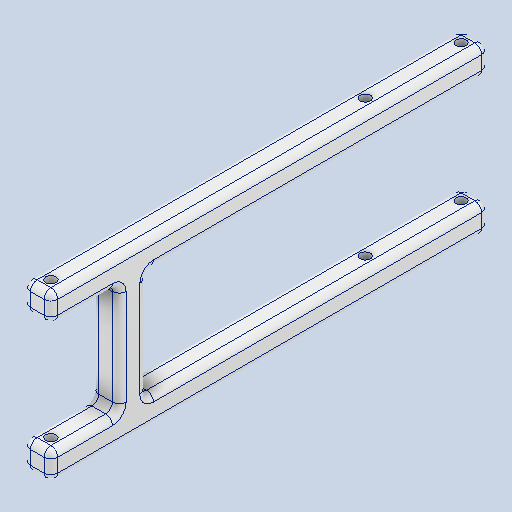
# Autodesk Inventor part: inner swing
Saved by Autodesk Inventor 2023 (Build 270158000, 158)
## iProperties
Created: 2023-01-25
Part Number: inner swing
Material: Aluminum 6061
Document SubType Name: Modeling
Designer: Gabriel - T3 CAD
Density: 2.7 g/cm^3
Appearance: Aluminum - Flat
Mass: 184.405 g
Surface Area: 217.239 cm^2
Volume: 68.2983 cm^3
Author: Gabriel - T3 CAD
Autodesk Inventor part; units mm, degrees
ref_plane "YZ Plane" through (0, 0, 0) normal (1, 0, 0) x (0, 1, 0)
ref_plane "XZ Plane" through (0, 0, 0) normal (0, 1, 0) x (-1, 0, 0)
ref_plane "XY Plane" through (0, 0, 0) normal (0, 0, 1) x (1, 0, 0)
sketch "Sketch1" plane through (0, 0, 0) normal (0, 1, 0) x (-1, 0, 0)
  line L0 (0, 0) -> (12.7, 0)
  line L1 (12.7, 0) -> (12.7, 203.2)
  line L2 (12.7, 203.2) -> (0, 203.2)
  line L3 (0, 203.2) -> (0, 0)
  circle A0 centre (6.35, 6.35) radius 2.3813
  circle A1 centre (6.35, 196.85) radius 2.3813
  circle A2 centre (6.35, 50.8) radius 2.3813
  dimension "d0" = 12.7
  dimension "d1" = 203.2
  dimension "d2" = 6.35
  dimension "d3" = 6.35
  dimension "d4" = 4.7625
  dimension "d5" = 6.35
  dimension "d6" = 4.7625
  dimension "d7" = 6.35
  dimension "d19" = 4.7625
  dimension "d20" = 6.35
  dimension "d21" = 50.8
  constraints: 8 end point, 3 centre point, 2 parallel, 1 horizontal, 1 perpendicular
  measures "d0" distance of L2.end L1.end
  measures "d1" distance of L1.end L0.end
  measures "d2" distance from line of L0 A0.centre
  measures "d3" distance from line of L1 A0.centre
  measures "d4" diameter of A0
  measures "d5" distance from line of L1 A1.centre
  measures "d6" diameter of A1
  measures "d7" distance from line of L2 A1.centre
  measures "d19" diameter of A2
  measures "d20" distance from line of L1 A2.centre
  measures "d21" distance from line of L0 A2.centre
extrude "Extrusion1" add sketch "Sketch1" along normal blind 76.2
sketch "Sketch2" plane through (0, 0, 203.2) normal (1, 0, 0) x (0, 0, -1)
  line L0 (203.2, 76.2) -> (0, 76.2) projected
  line L1 (0, 76.2) -> (31.75, 76.2)
  line L2 (31.75, 76.2) -> (31.75, 0)
  line L3 (31.75, 0) -> (0, 0)
  line L4 (0, 0) -> (0, 76.2)
  line L5 (203.2, 76.2) -> (177.8, 76.2)
  line L6 (177.8, 76.2) -> (177.8, 0)
  line L7 (177.8, 0) -> (203.2, 0)
  line L8 (203.2, 0) -> (203.2, 76.2)
  line L9 (203.2, 0) -> (203.2, 76.2) projected
  line L10 (203.2, 63.5) -> (0, 63.5)
  line L11 (0, 63.5) -> (0, 12.7)
  line L12 (0, 12.7) -> (203.2, 12.7)
  line L13 (203.2, 12.7) -> (203.2, 63.5)
  line L14 (0, 0) -> (203.2, 0) projected
  line L15 (31.75, 63.5) -> (44.45, 63.5)
  line L16 (44.45, 63.5) -> (44.45, 12.7)
  line L17 (44.45, 12.7) -> (31.75, 12.7)
  line L18 (31.75, 12.7) -> (31.75, 63.5)
  line L19 (177.8, 63.5) -> (165.1, 63.5)
  line L20 (165.1, 12.7) -> (177.8, 12.7)
  line L21 (177.8, 12.7) -> (177.8, 63.5)
  line L22 (139.7, 63.5) -> (139.7, 12.7)
  line L23 (139.7, 63.5) -> (127, 63.5)
  line L24 (127, 63.5) -> (127, 12.7)
  line L25 (127, 12.7) -> (139.7, 12.7)
  line L26 (139.7, 12.7) -> (139.7, 63.5)
  point P0 (177.8, 12.7)
  point P1 (184.15, 63.5)
  point P2 (0, 12.7)
  point P3 (31.75, 12.7)
  point P4 (19.05, 63.5)
  point P5 (0, 63.5)
  point P6 (44.45, 63.5)
  point P7 (31.75, 12.7)
  dimension "d10" = 31.75
  dimension "d12" = 25.4
  dimension "d13" = 76.2
  dimension "d14" = 203.2
  dimension "d15" = 50.8
  dimension "d16" = 12.7
  dimension "d22" = 12.7
  dimension "d24" = 63.5
  dimension "d25" = 12.7
  constraints: 48 end point, 11 parallel, 10 point on line, 6 horizontal, 6 perpendicular
  measures "d10" distance of L2.end L3.end
  measures "d12" distance of L7.end L6.end
  measures "d13" distance of L6.end L5.end
  measures "d14" distance of L12.end L11.end
  measures "d15" distance of L11.end L10.end
  measures "d16" distance between parallel lines of L14 L12
  measures "d22" distance of L16.end L17.end
  measures "d24" distance between parallel lines of L8 L22
  measures "d25" distance of L25.end L24.end
extrude "Extrusion2" cut sketch "Sketch2" against normal blind 12.7 contours L8 L12 L6 L10 | L6 L12 L22 L10 | L2 L12 L4 L10 | L10 L24 L12 L16 | L22 L12 L24 L10
fillet "Fillet1" radius 3.175 36 edges at (0, 38.1, 158.75) (0, 38.1, 171.45) (-12.7, 38.1, 171.45) (-12.7, 38.1, 158.75) (0, 63.5, 79.375) (0, 76.2, 101.6) (-12.7, 76.2, 101.6) (-12.7, 63.5, 79.375) (0, 63.5, 187.325) (-12.7, 63.5, 187.325) (-6.35, 63.5, 158.75) (-6.35, 63.5, 171.45) (-12.7, 12.7, 79.375) (0, 12.7, 79.375) (-12.7, 0, 101.6) (0, 0, 101.6) (0, 12.7, 187.325) (-12.7, 12.7, 187.325) (-6.35, 12.7, 171.45) (-6.35, 12.7, 158.75) (-6.35, 12.7, 203.2) (0, 6.35, 203.2) (-6.35, 0, 203.2) (-12.7, 6.35, 203.2) (0, 6.35, 0) (-6.35, 0, 0) (-12.7, 6.35, 0) (-6.35, 12.7, 0) (-6.35, 76.2, 0) (0, 69.85, 0) (-6.35, 63.5, 0) (-12.7, 69.85, 0) (0, 69.85, 203.2) (-6.35, 63.5, 203.2) (-12.7, 69.85, 203.2) (-6.35, 76.2, 203.2)
body "Solid1"
